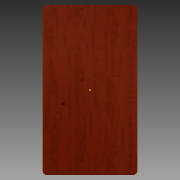
# Autodesk Inventor part: base-frame
Saved by Autodesk Inventor 2015 (Build 190159000, 159)
## iProperties
Created: 2014-07-15
Part Number: base-frame
Material: Wood (Oak)
Document SubType Name: Modeling
Designer: pc
Density: 0.76 g/cm^3
Appearance: White Oak - Natural Medium Gloss
d56: 44.000 mm
wallw: 42.000 mm
wall1_thick: 8.000 mm
wall2_thick: 6.400 mm
wall3_thick: 4.000 mm
wall1slot: 8.120 mm
wall2slot: 6.520 mm
wall3slot: 4.120 mm
gap1: 30.000 mm
gap2: 28.000 mm
baseh: 79.120 mm
basew: 44.000 mm
base_thick: 6.000 mm
base_slots_depth: 4.000 mm
d57: 79.120 mm
printer3dtolerance: 0.120 mm
wallh: 44.000 mm
cornerrad: 2.000 mm
baseextra: 2.000 mm
d80: 30.000 mm
d60: 6.000 mm
d62: 8.120 mm
d61: 0.00 deg
d91: 2.000 mm
d90: 2.000 mm
d89: 2.000 mm
d88: 2.000 mm
d87: 0.00 deg
d86: 4.000 mm
d84: 42.000 mm
d83: 4.120 mm
d82: 0.00 deg
d81: 4.000 mm
d79: 0.00 deg
d78: 4.000 mm
d77: 1.000 mm
d76: 42.000 mm
d75: 6.520 mm
d66: 1.000 mm
d64: 42.000 mm
d63: 1.000 mm
Author: pc
Autodesk Inventor part; units mm, degrees
ref_plane "YZ Plane" through (0, 0, 0) normal (1, 0, 0) x (0, 1, 0)
ref_plane "XZ Plane" through (0, 0, 0) normal (0, 1, 0) x (-1, 0, 0)
ref_plane "XY Plane" through (0, 0, 0) normal (0, 0, 1) x (1, 0, 0)
sketch "Base" plane through (0, 0, 0) normal (0, 0, 1) x (1, 0, 0)
  line L0 (-22, -39.56) -> (22, -39.56)
  line L1 (22, -39.56) -> (22, 39.56)
  line L2 (22, 39.56) -> (-22, 39.56)
  line L3 (-22, 39.56) -> (-22, -39.56)
  line L4 (-22, -39.56) -> (22, 39.56) construction
  line L5 (22, -39.56) -> (-22, 39.56) construction
  point P0 (0, 0)
  dimension "d56" = 44
  dimension "d57" = 79.12
  constraints: 12 end point, 2 midpoint, 2 parallel, 1 horizontal, 1 perpendicular
  measures "d56" distance of L0.start L0.end
  measures "d57" distance of L2.end L0.start
extrude "Extrusion4" add sketch "Base" along normal blind 6
sketch "Slot1" plane through (0, 0, 6) normal (0, 0, 1) x (1, 0, 0)
  line L0 (21, -38.56) -> (-21, -38.56)
  line L1 (-21, -38.56) -> (-21, -30.44)
  line L2 (-21, -30.44) -> (21, -30.44)
  line L3 (21, -30.44) -> (21, -38.56)
  line L4 (21, -38.56) -> (-21, -30.44) construction
  line L5 (-21, -38.56) -> (21, -30.44) construction
  line L6 (22, -39.56) -> (22, 39.56) projected
  line L7 (-22, -39.56) -> (22, -39.56) projected
  point P0 (0, 0)
  point P1 (0, -34.5)
  dimension "d62" = 8.12
  dimension "d63" = 1
  dimension "d64" = 42
  dimension "d66" = 1
  constraints: 12 end point, 2 midpoint, 2 parallel, 1 horizontal, 1 perpendicular
  measures "d62" distance of L0.end L1.end
  measures "d63" distance between parallel lines of L6 L3
  measures "d64" distance of L0.start L0.end
  measures "d66" distance between parallel lines of L7 L0
extrude "Slot1 slot" cut sketch "Slot1" against normal blind 4
sketch "Slot2" plane through (0, 0, 6) normal (0, 0, 1) x (1, 0, 0)
  line L0 (21, -0.44) -> (-21, -0.44)
  line L1 (-21, -0.44) -> (-21, 6.08)
  line L2 (-21, 6.08) -> (21, 6.08)
  line L3 (21, 6.08) -> (21, -0.44)
  line L4 (21, -0.44) -> (-21, 6.08) construction
  line L5 (-21, -0.44) -> (21, 6.08) construction
  line L6 (-22, 39.56) -> (-22, -39.56) projected
  line L7 (-21, -30.44) -> (21, -30.44) projected
  point P0 (0, 0)
  point P1 (0, 2.82)
  dimension "d75" = 6.52
  dimension "d76" = 42
  dimension "d77" = 1
  dimension "d80" = 30
  constraints: 12 end point, 2 midpoint, 2 parallel, 1 horizontal, 1 perpendicular
  measures "d75" distance of L0.end L1.end
  measures "d76" distance of L0.start L0.end
  measures "d77" distance between parallel lines of L6 L1
  measures "d80" distance between parallel lines of L7 L0
extrude "Slot2 slot" cut sketch "Slot2" against normal blind 4
sketch "Slot3" plane through (0, 0, 6) normal (0, 0, 1) x (1, 0, 0)
  line L0 (-21, 38.2) -> (21, 38.2)
  line L1 (21, 38.2) -> (21, 34.08)
  line L2 (21, 34.08) -> (-21, 34.08)
  line L3 (-21, 34.08) -> (-21, 38.2)
  line L4 (-21, 38.2) -> (21, 34.08) construction
  line L5 (21, 38.2) -> (-21, 34.08) construction
  point P0 (0, 36.14)
  dimension "d83" = 4.12
  dimension "d84" = 42
  constraints: 12 end point, 2 midpoint, 2 parallel, 1 horizontal, 1 perpendicular
  measures "d83" distance of L2.end L0.start
  measures "d84" distance of L0.start L0.end
extrude "Extrusion7" cut sketch "Slot3" against normal blind 4
fillet "Fillet1" radius 2 1 edges at (-22, 39.56, 3)
fillet "Fillet2" radius 2 1 edges at (22, 39.56, 3)
fillet "Fillet3" radius 2 1 edges at (22, -39.56, 3)
fillet "Fillet4" radius 2 1 edges at (-22, -39.56, 3)
sketch "Sketch14" plane through (0, 0, 6) normal (0, 0, 1) x (1, 0, 0)
  point P0 (0, 0)
equation "\"d56\" = basew"
equation "\"d57\" = baseh"
equation "\"d62\" = wall1slot"
equation "\"d63\" = -0.5 * wallw + 0.5 * basew"
equation "\"d64\" = wallw"
equation "\"d66\" = 0.5 * baseextra"
equation "\"d75\" = wall2slot"
equation "\"d76\" = wallw"
equation "\"d77\" = 0.5 * baseextra"
equation "\"d80\" = gap1"
equation "\"d83\" = wall3slot"
equation "\"d84\" = wallw"
equation "\"printer3dtolerance\" = 0.12"
equation "\"wallw\" = 42"
equation "\"wallh\" = 44"
equation "\"cornerrad\" = 2"
equation "\"baseextra\" = 2"
equation "\"wall1_thick\" = 8"
equation "\"wall2_thick\" = 6.4"
equation "\"wall3_thick\" = 4"
equation "\"wall1slot\" = 8.12"
equation "\"wall2slot\" = 6.52"
equation "\"wall3slot\" = 4.12"
equation "\"gap1\" = 30"
equation "\"gap2\" = 28"
equation "\"baseh\" = 79.12"
equation "\"basew\" = 44"
equation "\"base_thick\" = 6"
equation "\"base_slots_depth\" = 4"
equation "\"d26\" = 8.12"
equation "\"d27\" = 42"
equation "\"d28\" = 44"
equation "\"d29\" = 28"
equation "\"d31\" = 4.12"
equation "\"d32\" = 6.52"
equation "\"d33\" = 79.12"
equation "\"d39\" = 8.12"
equation "\"d40\" = 42"
equation "\"d41\" = 44"
equation "\"d48\" = 8.12"
equation "\"d49\" = 42"
equation "\"d50\" = 8.12"
equation "\"d51\" = 42"
equation "\"d52\" = 44"
equation "\"d53\" = 44"
equation "\"d71\" = 8.12"
equation "\"d72\" = 42"
equation "\"d73\" = 2"
equation "\"d74\" = 44"
equation "\"distancefrombottom\" = 34"
equation "\"servosmallcircledia\" = 5.92"
equation "\"servo9gw\" = 22.8"
equation "\"servomountsquare\" = 6"
equation "\"servopolygonl\" = 5.92"
equation "\"servopolygonr\" = 6.12"
equation "\"distancefromleft\" = 26"
equation "\"servobigcircledia\" = 11.62"
equation "\"servomounth\" = 4"
equation "\"wall3slotd\" = 2"
equation "\"wall3slotw\" = 36"
equation "\"adapterh\" = 16"
equation "\"adapterw\" = 32"
equation "\"wall3slotd_1\" = 2"
body "Solid2"
